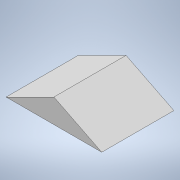
# Autodesk Inventor part: houseDormerRoof
Saved by Autodesk Inventor 2022 (Build 260153070, 153G)
## iProperties
Created: 2021-07-13
Part Number: houseDormerRoof
Material: Generic
Document SubType Name: Modeling
Designer: robst
Density: 1 g/cm^3
Appearance: Default
Author: robst
Autodesk Inventor part; units mm, degrees
ref_plane "YZ Plane" through (0, 0, 0) normal (1, 0, 0) x (0, 1, 0)
ref_plane "XZ Plane" through (0, 0, 0) normal (0, 1, 0) x (-1, 0, 0)
ref_plane "XY Plane" through (0, 0, 0) normal (0, 0, 1) x (1, 0, 0)
sketch "Sketch1" plane through (0, 0, 0) normal (0, 0, 1) x (1, 0, 0)
  line L0 (0, 0) -> (0, 1885.628) construction
  line L1 (0, 1885.628) -> (-3771.2645, 0)
  line L2 (-3771.2645, 0) -> (0, 0)
  line L3 (0, 0) -> (3771.2645, 0)
  line L4 (0, 1885.628) -> (3771.2645, 0)
  dimension "d0" = 26.565
  dimension "d1" = 4216.4
  dimension "d2" = 26.565
  dimension "d3" = 4216.4
  constraints: 10 end point, 2 horizontal, 1 vertical
  measures "d0" angle of L1 L2
  measures "d1" distance of L0.end L1.end
  measures "d2" angle of L3 L4
  measures "d3" distance of L0.end L3.end
extrude "Extrusion1" add sketch "Sketch1" against normal blind 5689.6
equation "\"d2\" = pitch_6_12"
equation "\"pitch_6_12\" = 26.565deg"
body "Solid1"
